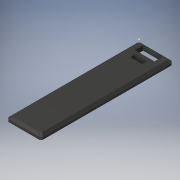
# Autodesk Inventor part: Battery-Management-Case-Cover
Saved by Autodesk Inventor 2019 (Build 230136000, 136)
## iProperties
Created: 2018-12-05
Part Number: Battery-Management-Case-Cover
Material: Generic
Document SubType Name: Modeling
Designer: lateSWE
Density: 1 g/cm^3
Appearance: Default
Author: lateSWE
Autodesk Inventor part; units mm, degrees
ref_plane "YZ Plane" through (0, 0, 0) normal (1, 0, 0) x (0, 1, 0)
ref_plane "XZ Plane" through (0, 0, 0) normal (0, 1, 0) x (-1, 0, 0)
ref_plane "XY Plane" through (0, 0, 0) normal (0, 0, 1) x (1, 0, 0)
sketch "Sketch1" plane through (0, 0, 0) normal (0, 0, 1) x (1, 0, 0)
  line L0 (0, 0) -> (22.5, 0)
  line L1 (22.5, 0) -> (22.5, 3)
  line L2 (22.5, 3) -> (0, 3)
  line L3 (0, 3) -> (0, 0)
  dimension "d0" = 22.5
  dimension "d1" = 3
  constraints: 8 end point, 2 parallel, 1 horizontal, 1 perpendicular
  measures "d0" distance of L2.end L1.end
  measures "d1" distance of L1.end L0.end
extrude "Extrusion1" add sketch "Sketch1" along normal blind 86.75
sketch "Sketch2" plane through (0, 3, 0) normal (0, 1, 0) x (1, 0, 0)
  line L0 (0, 0) -> (22.5, 0) projected
  line L1 (11.25, 0) -> (11.25, -2)
  line L2 (11.25, 0) -> (13.25, 0) construction
  line L3 (11.25, -2) -> (4.75, -2)
  line L4 (4.75, -2) -> (4.75, -7.5)
  line L5 (4.75, -7.5) -> (11.25, -7.5)
  line L6 (11.25, -7.5) -> (11.25, -2)
  line L7 (11.25, -2) -> (17.75, -2)
  line L8 (17.75, -2) -> (17.75, -7.5)
  line L9 (17.75, -7.5) -> (11.25, -7.5)
  line L10 (11.25, -7.5) -> (11.25, -2)
  dimension "d4" = 2
  dimension "d5" = 90
  dimension "d6" = 6.5
  dimension "d7" = 5.5
  dimension "d8" = 6.5
  dimension "d9" = 5.5
  constraints: 20 end point, 4 parallel, 3 horizontal, 3 perpendicular, 1 midpoint, 1 vertical
  measures "d4" distance of L1.start L1.end
  measures "d5" angle of L1 L2
  measures "d6" distance of L5.end L4.end
  measures "d7" distance of L4.end L3.end
  measures "d8" distance of L8.end L9.end
  measures "d9" distance of L7.end L8.end
extrude "Extrusion2" cut sketch "Sketch2" against normal blind 3
sketch "Sketch3" plane through (0, 3, 0) normal (0, 1, 0) x (1, 0, 0)
  line L0 (4.75, -7.5) -> (17.75, -7.5) projected
  line L1 (11.25, -7.5) -> (11.25, -10)
  line L2 (11.25, -7.5) -> (13.75, -7.5) construction
  line L3 (11.25, -10) -> (7.25, -10)
  line L4 (7.25, -10) -> (7.25, -13)
  line L5 (7.25, -13) -> (11.25, -13)
  line L6 (11.25, -13) -> (11.25, -10)
  line L7 (11.25, -10) -> (15.25, -10)
  line L8 (15.25, -10) -> (15.25, -13)
  line L9 (15.25, -13) -> (11.25, -13)
  line L10 (11.25, -13) -> (11.25, -10)
  point P0 (0, 0)
  dimension "d12" = 2.5
  dimension "d13" = 90
  dimension "d14" = 4
  dimension "d15" = 3
  dimension "d16" = 4
  dimension "d17" = 3
  constraints: 20 end point, 4 parallel, 3 horizontal, 3 perpendicular, 1 midpoint, 1 vertical
  measures "d12" distance of L1.start L1.end
  measures "d13" angle of L1 L2
  measures "d14" distance of L5.end L4.end
  measures "d15" distance of L4.end L3.end
  measures "d16" distance of L8.end L9.end
  measures "d17" distance of L7.end L8.end
extrude "Extrusion3" cut sketch "Sketch3" against normal blind 3
sketch "Sketch4" plane through (0, 3, 0) normal (0, 1, 0) x (1, 0, 0)
  point P0 (0, 0)
chamfer "Chamfer1" distance 1.5 angle 45 4 edges at (22.5, 3, 43.375) (11.25, 3, 86.75) (0, 3, 43.375) (11.25, 3, 0)
chamfer "Chamfer2" distance 1 angle 45 4 edges at (0, 0.75, 86.75) (22.5, 0.75, 86.75) (22.5, 0.75, 0) (0, 0.75, 0)
chamfer "Chamfer3" distance 0.8165 angle 45 4 edges at (1, 2.5, 1) (21.5, 2.5, 1) (1, 2.5, 85.75) (21.5, 2.5, 85.75)
body "Solid1"
